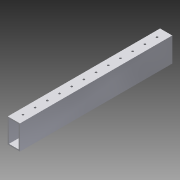
# Autodesk Inventor part: VersaFrame Side Rail
Saved by Autodesk Inventor 2015 (Build 190159000, 159)
## iProperties
Created: 2014-12-18
Part Number: VersaFrame Side Rail
Material: Aluminum 6061
Document SubType Name: Modeling
Designer: Nemo
Density: 2.7 g/cm^3
Appearance: Aluminum - Flat
Length: 12.500 in
HoleOffset: 0.500 in
Author: Nemo
Autodesk Inventor part; units mm, degrees
ref_plane "YZ Plane" through (0, 0, 0) normal (1, 0, 0) x (0, 1, 0)
ref_plane "XZ Plane" through (0, 0, 0) normal (0, 1, 0) x (-1, 0, 0)
ref_plane "XY Plane" through (0, 0, 0) normal (0, 0, 1) x (1, 0, 0)
sketch "Sketch1" plane through (0, 0, 0) normal (0, 0, 1) x (1, 0, 0)
  line L0 (12.7, -25.4) -> (-12.7, -25.4)
  line L1 (-12.7, -25.4) -> (-12.7, 25.4)
  line L2 (-12.7, 25.4) -> (12.7, 25.4)
  line L3 (12.7, 25.4) -> (12.7, -25.4)
  line L4 (12.7, -25.4) -> (-12.7, 25.4) construction
  line L5 (-12.7, -25.4) -> (12.7, 25.4) construction
  line L6 (10.16, 22.86) -> (-10.16, 22.86)
  line L7 (-10.16, 22.86) -> (-10.16, -22.86)
  line L8 (-10.16, -22.86) -> (10.16, -22.86)
  line L9 (10.16, -22.86) -> (10.16, 22.86)
  point P0 (0, 0)
  dimension "d0" = 25.4
  dimension "d1" = 50.8
  dimension "d2" = 2.54
  constraints: 20 end point, 4 parallel, 2 midpoint, 2 perpendicular, 1 horizontal, 3 other
  measures "d0" distance of L1.end L2.end
  measures "d1" distance of L0.end L1.end
  measures "d2" distance between parallel lines of L2 L6
extrude "Extrusion1" add sketch "Sketch1" along normal mid plane 317.5
sketch "Sketch2" plane through (-12.7, 25.4, 158.75) normal (0, 1, 0) x (1, 0, 0)
  point P0 (12.7, 158.75)
  point P1 (12.7, 171.45)
  point P2 (12.7, 146.05)
  dimension "HoleOffset" = 12.7
  dimension "d6" = 12.7
  constraints: 2 vertical alignment
  measures "HoleOffset" distance of point (12.7, 158.75) point (12.7, 171.45)
  measures "d6" distance of point (12.7, 158.75) point (12.7, 146.05)
hole "Hole1" at (0, 25.4, -12.7) at (0, 25.4, 12.7) direction (0, -1, 0) diameter 4.1656 end through all
pattern_linear "Rectangular Pattern1" count 31 spacing 50.8 along (0, 0, 1) of "Hole1" first direction both ways yes
body "Solid1"
